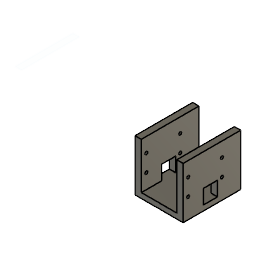
그리퍼_최종 (Autodesk Fusion 360 archive; units mm, degrees)
design "01.03 그리퍼-로봇팔 연결부위"
Autodesk Fusion 360 part; units mm, degrees
sketch "스케치1" plane through (0, 0, 21.6) normal (0, 0, 1) x (-1, 0, 0)
  line L0 (-16.75, -11.75) -> (-16.75, 42.75)
  line L1 (-16.75, 42.75) -> (-22.75, 42.75)
  line L2 (-22.75, 42.75) -> (-22.75, -11.75)
  line L3 (-22.75, -11.75) -> (-16.75, -11.75)
sketch "스케치2" plane through (0, 0, 21.6) normal (0, 0, 1) x (1, 0, 0)
sketch "스케치3" plane through (0, 0, 0) normal (1, 0, 0) x (0, 1, 0)
  line L0 (-42.75, 21.6) -> (11.75, 21.6)
  line L1 (11.75, 21.6) -> (11.75, -17)
  line L2 (11.75, -17) -> (-42.75, -17)
  line L3 (-42.75, -17) -> (-42.75, 21.6)
  circle A0 centre (-38, 8) radius 1.35
  circle A1 centre (-6, 8) radius 1.35
  circle A2 centre (-6, -8) radius 1.35
  circle A3 centre (-38, -8) radius 1.35
  line L4 (-23.5, -8.4) -> (-10.3, -8.4)
  line L5 (-10.3, -8.4) -> (-10.3, -17)
  line L6 (-10.3, -17) -> (-23.5, -17)
  line L7 (-23.5, -17) -> (-23.5, -8.4)
  line L8 (11.75, -17) -> (-42.75, -17)
  line L9 (-42.75, -17) -> (-42.75, -22)
  line L10 (-42.75, -22) -> (11.75, -22)
  line L11 (11.75, -22) -> (11.75, -17)
  dimension "d1" = 2.7
  dimension "d2" = 2.7
  dimension "d3" = 2.7
  dimension "d4" = 2.7
  constraint horizontal L0
  constraint vertical L1
  constraint horizontal L2
  constraint vertical L3
  constraint horizontal L4
  constraint vertical L5
  constraint horizontal L6
  constraint vertical L7
  constraint coincident L2 L5.end
  constraint horizontal L8
  constraint vertical L9
  constraint horizontal L10
  constraint vertical L11
  measures "d1" diameter of A0
  measures "d2" diameter of A1
  measures "d3" diameter of A2
  measures "d4" diameter of A3
extrude "돌출1" add sketch "스케치3" along normal blind 6 contours L0 L1 L2 L3 L4 L5 L7 L8 | L2 L6 L8 L9 L10 L11 makes body 1
move_body "이동1" bodies 1 to x (1, 0, 0) y (0, 1, 0) z (0, 0, 1) at (130, 0, 0)
sketch "스케치4" plane through (136, 0, 0) normal (1, 0, 0) x (0, 1, 0)
  circle A0 centre (-6, -8) radius 1.35
  circle A1 centre (-38, 8) radius 1.35
  line L0 (-23.5, -8.4) -> (-10.3, -8.4)
  line L1 (-10.3, -8.4) -> (-10.3, -17)
  line L2 (-10.3, -17) -> (-23.5, -17)
  line L3 (-23.5, -17) -> (-23.5, -8.4)
  circle A2 centre (-6, 8) radius 1.35
  circle A3 centre (-38, -8) radius 1.35
  line L4 (-42.75, 21.6) -> (-42.75, -22)
  line L5 (-42.75, -22) -> (11.75, -22)
  line L6 (11.75, -22) -> (11.75, 21.6)
  line L7 (11.75, 21.6) -> (-42.75, 21.6)
  line L8 (-10.3, -17) -> (-23.5, -17)
  line L9 (-23.5, -17) -> (-23.5, -22)
  line L10 (-23.5, -22) -> (-10.3, -22)
  line L11 (-10.3, -22) -> (-10.3, -17)
  constraint horizontal L8
  constraint vertical L9
  constraint horizontal L10
  constraint vertical L11
  constraint coincident L5 L9.end
  constraint coincident L1.end L2.start
sketch "스케치5" plane through (136, 0, 0) normal (1, 0, 0) x (0, 1, 0)
extrude "돌출2" cut sketch "스케치4" against normal blind 6 contours L2 L5 L8 L9 L10 L11 bodies 1
copy_body "본체 복사하여 붙여넣기1" bodies 1 makes body 2
move_body "이동2" bodies 2 to x (1, 0, 0) y (0, 1, 0) z (0, 0, 1) at (33.5, 0, 0)
move_body "이동3" bodies 2 to x (1, 0, 0) y (0, 1, 0) z (0, 0, 1) at (6, 0, 0)
sketch "스케치6" plane through (0, 0, 0) normal (0, 0, 1) x (1, 0, 0)
  line L0 (130, -42.75) -> (175.5, -42.75)
  line L1 (175.5, -42.75) -> (175.5, 11.75)
  line L2 (175.5, 11.75) -> (130, 11.75)
  line L3 (130, 11.75) -> (130, -42.75)
  constraint horizontal L0
  constraint vertical L1
  constraint horizontal L2
  constraint vertical L3
extrude "돌출3" add sketch "스케치6" along normal blind -27 and the other way blind 22 bodies 1 2
sketch "스케치7" plane through (0, -42.75, 0) normal (0, -1, 0) x (1, 0, 0)
  line L0 (130, -27) -> (175.5, -27)
  line L1 (152.75, -27) -> (152.75, -38.961)
  circle A0 centre (152.75, -38.961) radius 12.15
  dimension "d13" = 11.961
  dimension "d14" = 24.3
  constraint midpoint L0 L1.start
  constraint perpendicular L0 L1
  constraint coincident L1.end A0.centre
  measures "d13" distance of L1.start L1.end
  measures "d14" diameter of A0
extrude "돌출4" cut sketch "스케치7" against normal blind 54.5 contours L0 A0 picked at (151.8001, -26.944) bodies 1
ref_plane "작업 평면1" through (152.75, -30.7254, -26.811) normal (0, 0, -1) x (1, 0, 0)
